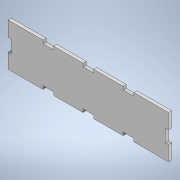
# Autodesk Inventor part: Стекнка t1
Saved by Autodesk Inventor 2021 (Build 250183000, 183)
## iProperties
Created: 2021-04-10
Part Number: Стекнка t1
Material: Типовые
Document SubType Name: Modeling
Designer: user
Density: 1 g/cm^3
Appearance: По умолчанию
Author: user
Autodesk Inventor part; units mm, degrees
ref_plane "YZ Plane" through (0, 0, 0) normal (1, 0, 0) x (0, 1, 0)
ref_plane "XZ Plane" through (0, 0, 0) normal (0, 1, 0) x (-1, 0, 0)
ref_plane "XY Plane" through (0, 0, 0) normal (0, 0, 1) x (1, 0, 0)
sketch "Эскиз1" plane through (0, 0, 0) normal (0, 0, 1) x (1, 0, 0)
  line L0 (-75, 6) -> (-75, 20)
  line L1 (-75, 20) -> (-42.5, 20)
  line L2 (-32.5, 20) -> (-32.5, 17)
  line L3 (-32.5, 17) -> (-42.5, 17)
  line L4 (-42.5, 17) -> (-42.5, 20)
  line L5 (-32.5, 20) -> (-5, 20)
  line L6 (0, 17) -> (-5, 17)
  line L7 (-5, 17) -> (-5, 20)
  line L8 (-72, 0) -> (-72, 6)
  line L9 (-72, 6) -> (-75, 6)
  line L10 (-75, 20) -> (-42.5, 20)
  line L11 (-32.5, 20) -> (-5, 20)
  line L12 (75, 6) -> (75, 20)
  line L13 (75, 20) -> (42.5, 20)
  line L14 (32.5, 20) -> (32.5, 17)
  line L15 (32.5, 17) -> (42.5, 17)
  line L16 (42.5, 17) -> (42.5, 20)
  line L17 (32.5, 20) -> (5, 20)
  line L18 (0, 17) -> (5, 17)
  line L19 (5, 17) -> (5, 20)
  line L20 (72, 0) -> (72, 6)
  line L21 (72, 6) -> (75, 6)
  line L22 (75, 20) -> (42.5, 20)
  line L23 (32.5, 20) -> (5, 20)
  line L24 (-75, -6) -> (-75, -20)
  line L25 (-75, -20) -> (-42.5, -20)
  line L26 (-32.5, -20) -> (-32.5, -17)
  line L27 (-32.5, -17) -> (-42.5, -17)
  line L28 (-42.5, -17) -> (-42.5, -20)
  line L29 (-32.5, -20) -> (-5, -20)
  line L30 (0, -17) -> (-5, -17)
  line L31 (-5, -17) -> (-5, -20)
  line L32 (-72, 0) -> (-72, -6)
  line L33 (-72, -6) -> (-75, -6)
  line L34 (-75, -20) -> (-42.5, -20)
  line L35 (-32.5, -20) -> (-5, -20)
  line L36 (75, -6) -> (75, -20)
  line L37 (75, -20) -> (42.5, -20)
  line L38 (32.5, -20) -> (32.5, -17)
  line L39 (32.5, -17) -> (42.5, -17)
  line L40 (42.5, -17) -> (42.5, -20)
  line L41 (32.5, -20) -> (5, -20)
  line L42 (0, -17) -> (5, -17)
  line L43 (5, -17) -> (5, -20)
  line L44 (72, 0) -> (72, -6)
  line L45 (72, -6) -> (75, -6)
  line L46 (75, -20) -> (42.5, -20)
  line L47 (32.5, -20) -> (5, -20)
  point P0 (0, 0)
  constraints: 96 end point, 2 horizontal, 1 parallel
extrude "Выдавливание1" add sketch "Эскиз1" along normal blind 3
